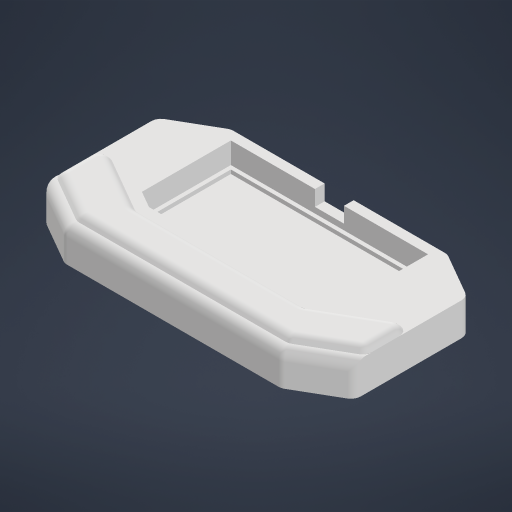
# Autodesk Inventor part: Joystick Bottom
Saved by Autodesk Inventor 2023.4 (Build 274418000, 418)
## iProperties
Created: 2024-04-17
Part Number: Joystick Bottom
Material: Generic
Document SubType Name: Modeling
Designer: xSibe
Density: 1 g/cm^3
Appearance: Default
Author: xSibe
Autodesk Inventor part; units mm, degrees
ref_plane "YZ Plane" through (0, 0, 0) normal (1, 0, 0) x (0, 1, 0)
ref_plane "XZ Plane" through (0, 0, 0) normal (0, 1, 0) x (-1, 0, 0)
ref_plane "XY Plane" through (0, 0, 0) normal (0, 0, 1) x (1, 0, 0)
sketch "Sketch1" plane through (0, 0, 0) normal (0, 1, 0) x (-1, 0, 0)
  line L0 (25.5, 11.5) -> (-25.5, 11.5)
  line L1 (-25.5, 11.5) -> (-25.5, -11.5)
  line L2 (-25.5, -11.5) -> (25.5, -11.5)
  line L3 (25.5, -11.5) -> (25.5, 11.5)
  line L4 (25.5, 11.5) -> (-25.5, -11.5) construction
  line L5 (-25.5, 11.5) -> (25.5, -11.5) construction
  line L6 (24.5, -10.5) -> (-24.5, -10.5)
  line L7 (-24.5, -10.5) -> (-24.5, 10.5)
  line L8 (-24.5, 10.5) -> (24.5, 10.5)
  line L9 (24.5, 10.5) -> (24.5, -10.5)
  line L10 (28, -14) -> (-28, -14)
  line L11 (-28, -14) -> (-28, 14)
  line L12 (-28, 14) -> (28, 14)
  line L13 (28, 14) -> (28, -14)
  line L14 (28, -14) -> (15.875644, -7)
  line L15 (15.875644, -7) -> (15.875644, 7)
  line L16 (15.875644, 7) -> (28, 14)
  line L17 (28, 14) -> (40.124356, 7)
  line L18 (40.124356, 7) -> (40.124356, -7)
  line L19 (40.124356, -7) -> (28, -14)
  line L20 (-28, -14) -> (-40.124356, -7)
  line L21 (-40.124356, -7) -> (-40.124356, 7)
  line L22 (-40.124356, 7) -> (-28, 14)
  line L23 (-28, 14) -> (-15.875644, 7)
  line L24 (-15.875644, 7) -> (-15.875644, -7)
  line L25 (-15.875644, -7) -> (-28, -14)
  line L26 (40.124356, 7) -> (40.124356, 22)
  line L27 (-28, 29) -> (28, 29)
  line L28 (-40.124356, 22) -> (-28, 29)
  line L29 (-40.124356, 22) -> (-40.124356, 7)
  line L30 (40.124356, 22) -> (28, 29)
  line L31 (28, 14) -> (28, 29)
  line L32 (-28, 14) -> (-28, 29)
  line L33 (-21.169873, 14) -> (21.169873, 14)
  line L34 (-25.5, 11.5) -> (-21.169873, 14)
  line L35 (25.5, 11.5) -> (21.169873, 14)
  point P0 (0, 0)
  point P1 (28, 0)
  point P2 (-28, 0)
  dimension "d0" = 51
  dimension "d1" = 23
  dimension "d2" = 1
  dimension "d3" = 2.5
  dimension "d13" = 15
  dimension "d20" = 15
  dimension "d21" = 90
  dimension "d22" = 60
  dimension "d23" = 150
  dimension "d24" = 150
  constraints: 72 end point, 7 parallel, 4 midpoint, 3 perpendicular, 3 vertical, 2 horizontal, 1 coincident, 1 collinear, 32 other
  measures "d0" distance of L2.end L1.end
  measures "d1" distance of L1.end L0.end
  measures "d2" distance between parallel lines of L2 L6
  measures "d3" distance between parallel lines of L2 L10
  measures "d13" distance of L17.end L26.end
  measures "d20" distance of L28.start L21.end
  measures "d21" angle of L31 L27
  measures "d22" angle of L28 L32
  measures "d23" angle of L33 L35
  measures "d24" angle of L34 L33
extrude "Extrusion1" add sketch "Sketch1" along normal blind 3
extrude "Extrusion2" cut sketch "Sketch1" against normal blind 1 from surface at 3 contours L16 L15 L14 L6 L25 L24 L23 L8 | L8 L9 L6 L14 L15 L16 | L23 L24 L25 L6 L7 L8
extrude "Extrusion3" add sketch "Sketch1" along normal blind 5.5 from surface at 3 contours L35 L16 L13 L14 L2 L3 | L35 L12 L16 | L14 L10 L25 L2 | L17 L18 L19 L13 | L31 L30 L26 L17 | L12 L32 L27 L31 | L1 L2 L25 L11 L23 L34 | L23 L12 L34 | L11 L20 L21 L22 | L22 L29 L28 L32
sketch "Sketch2" plane through (-28, 8.5, 14) normal (0, 1, 0) x (1, 0, 0)
  line L0 (2.5, 25.5) -> (2.5, 2.5)
  line L1 (53.5, 25.5) -> (2.5, 25.5)
  line L2 (53.5, 2.5) -> (53.5, 25.5)
  line L3 (0, 28) -> (56, 28)
  line L4 (53.5, 25.5) -> (53.5, 28)
  line L5 (2.5, 25.5) -> (2.5, 28)
  line L6 (2.5, 26.75) -> (53.5, 26.75)
  line L7 (24.25, 25.5) -> (31.75, 25.5)
  line L8 (31.75, 25.5) -> (31.75, 28)
  line L9 (31.75, 28) -> (24.25, 28)
  line L10 (24.25, 28) -> (24.25, 25.5)
  line L11 (24.25, 25.5) -> (31.75, 28) construction
  line L12 (31.75, 25.5) -> (24.25, 28) construction
  line L13 (68.124356, 21) -> (68.124356, -8)
  line L14 (56, 28) -> (68.124356, 21)
  line L15 (-12.124356, 21) -> (0, 28)
  line L16 (-12.124356, -8) -> (-12.124356, 21)
  line L17 (0, -15) -> (-12.124356, -8)
  line L18 (56, -15) -> (0, -15)
  line L19 (68.124356, -8) -> (56, -15)
  line L20 (6.830127, 0) -> (49.169873, 0)
  line L21 (2.5, 2.5) -> (6.830127, 0)
  line L22 (49.169873, 0) -> (53.5, 2.5)
  line L23 (53.5, 2.5) -> (2.5, 2.5)
  point P0 (28, 14)
  point P1 (28, 26.75)
  dimension "d10" = 7.5
  constraints: 20 end point, 5 midpoint, 3 perpendicular, 3 point on line, 2 horizontal, 2 parallel
  measures "d10" distance of L9.end L8.end
extrude "Extrusion4" cut sketch "Sketch2" against normal blind 4 contours L10 L6 L8 L1 | L10 L3 L8 L6
fillet "Fillet1" radius 2.5 11 edges at (-34.0622, 8.5, 25.5) (0, 8.5, 29) (34.0622, 8.5, 25.5) (40.1244, 4.25, 22) (28, 4.25, 29) (-28, 4.25, 29) (-40.1244, 4.25, 22) (-40.1244, 4.25, -7) (-28, 4.25, -14) (40.1244, 4.25, -7) (28, 4.25, -14)
extrude "Extrusion5" add sketch "Sketch2" along normal blind 3 from surface at -5.5 contours L23 L22 L20 L21
chamfer "Chamfer1" distance 1.675 angle 45 1 edges at (0, 6, 11.5)
sketch "Sketch3" plane through (-21.169873, 8.5, 14) normal (0, 1, 0) x (1, 0, 0)
  arc A0 (-1.25, -2.165064) -> (0, -2.5) centre (0, 0) ccw
  line L0 (0, -2.5) -> (42.339746, -2.5)
  arc A1 (42.339746, -2.5) -> (43.589746, -2.165064) centre (42.339746, 0) ccw
  line L1 (43.589746, -2.165064) -> (60.044229, 7.334936)
  arc A2 (60.044229, 7.334936) -> (61.294229, 9.5) centre (58.794229, 9.5) ccw
  line L2 (61.294229, 9.5) -> (61.294229, 19.556624)
  arc A3 (61.294229, 19.556624) -> (60.044229, 21.721688) centre (58.794229, 19.556624) ccw
  line L3 (60.044229, 21.721688) -> (49.75, 27.665064)
  arc A4 (49.75, 27.665064) -> (48.5, 28) centre (48.5, 25.5) ccw
  line L4 (48.5, 28) -> (-6.160254, 28)
  arc A5 (-6.160254, 28) -> (-7.410254, 27.665064) centre (-6.160254, 25.5) ccw
  line L5 (-7.410254, 27.665064) -> (-17.704483, 21.721688)
  arc A6 (-17.704483, 21.721688) -> (-18.954483, 19.556624) centre (-16.454483, 19.556624) ccw
  line L6 (-18.954483, 19.556624) -> (-18.954483, 9.5)
  arc A7 (-18.954483, 9.5) -> (-17.704483, 7.334936) centre (-16.454483, 9.5) ccw
  line L7 (-17.704483, 7.334936) -> (-1.25, -2.165064)
  line L8 (0.169873, 23.5) -> (42.169873, 23.5)
  arc A8 (44.669873, 21) -> (42.169873, 23.5) centre (42.169873, 21) ccw
  line L9 (44.669873, 21) -> (44.669873, 5.098076)
  arc A9 (43.419873, 2.933013) -> (44.669873, 5.098076) centre (42.169873, 5.098076) ccw
  line L10 (43.419873, 2.933013) -> (42.383975, 2.334936)
  arc A10 (41.133975, 2) -> (42.383975, 2.334936) centre (41.133975, 4.5) ccw
  line L11 (41.133975, 2) -> (28.044873, 2)
  arc A11 (-0.044229, 2.334936) -> (1.205771, 2) centre (1.205771, 4.5) ccw
  line L12 (-0.044229, 2.334936) -> (-1.080127, 2.933013)
  arc A12 (-2.330127, 5.098076) -> (-1.080127, 2.933013) centre (0.169873, 5.098076) ccw
  line L13 (-2.330127, 5.098076) -> (-2.330127, 21)
  arc A13 (0.169873, 23.5) -> (-2.330127, 21) centre (0.169873, 21) ccw
  arc A14 (49.75, 27.665064) -> (48.5, 28) centre (48.5, 25.5) ccw
  line L14 (60.044229, 21.721688) -> (49.75, 27.665064)
  arc A15 (61.294229, 19.556624) -> (60.044229, 21.721688) centre (58.794229, 19.556624) ccw
  line L15 (61.294229, -6.556624) -> (61.294229, 19.556624)
  arc A16 (60.044229, -8.721688) -> (61.294229, -6.556624) centre (58.794229, -6.556624) ccw
  line L16 (49.75, -14.665064) -> (60.044229, -8.721688)
  arc A17 (48.5, -15) -> (49.75, -14.665064) centre (48.5, -12.5) ccw
  line L17 (-6.160254, -15) -> (48.5, -15)
  arc A18 (-7.410254, -14.665064) -> (-6.160254, -15) centre (-6.160254, -12.5) ccw
  line L18 (-17.704483, -8.721688) -> (-7.410254, -14.665064)
  arc A19 (-18.954483, -6.556624) -> (-17.704483, -8.721688) centre (-16.454483, -6.556624) ccw
  line L19 (-18.954483, 19.556624) -> (-18.954483, -6.556624)
  arc A20 (-17.704483, 21.721688) -> (-18.954483, 19.556624) centre (-16.454483, 19.556624) ccw
  line L20 (-7.410254, 27.665064) -> (-17.704483, 21.721688)
  arc A21 (-6.160254, 28) -> (-7.410254, 27.665064) centre (-6.160254, 25.5) ccw
  line L21 (48.5, 28) -> (-6.160254, 28)
  line L22 (42.339746, -2.75) -> (0, -2.75)
  arc A22 (-1.375, -2.38157) -> (0, -2.75) centre (0, 0) ccw
  line L23 (-1.375, -2.38157) -> (-17.829483, 7.11843)
  arc A23 (-19.204483, 9.5) -> (-17.829483, 7.11843) centre (-16.454483, 9.5) ccw
  line L24 (-19.204483, 9.5) -> (-19.204483, 19.556624)
  arc A24 (-17.829483, 21.938194) -> (-19.204483, 19.556624) centre (-16.454483, 19.556624) ccw
  line L25 (-17.829483, 21.938194) -> (-7.535254, 27.88157)
  arc A25 (-6.160254, 28.25) -> (-7.535254, 27.88157) centre (-6.160254, 25.5) ccw
  line L26 (-6.160254, 28.25) -> (48.5, 28.25)
  arc A26 (49.875, 27.88157) -> (48.5, 28.25) centre (48.5, 25.5) ccw
  line L27 (49.875, 27.88157) -> (60.169229, 21.938194)
  arc A27 (61.544229, 19.556624) -> (60.169229, 21.938194) centre (58.794229, 19.556624) ccw
  line L28 (61.544229, 19.556624) -> (61.544229, 9.5)
  arc A28 (60.169229, 7.11843) -> (61.544229, 9.5) centre (58.794229, 9.5) ccw
  line L29 (60.169229, 7.11843) -> (43.714746, -2.38157)
  arc A29 (42.339746, -2.75) -> (43.714746, -2.38157) centre (42.339746, 0) ccw
  arc A30 (49.75, 27.665064) -> (48.5, 28) centre (48.5, 25.5) ccw
  line L30 (24.919873, 28) -> (48.5, 28)
  line L31 (24.919873, 28) -> (24.919873, 25.5)
  line L32 (46.669873, 25.5) -> (24.919873, 25.5)
  line L33 (46.669873, 2.5) -> (46.669873, 25.5)
  line L34 (42.339746, 0) -> (46.669873, 2.5)
  line L35 (0, 0) -> (42.339746, 0)
  line L36 (-4.330127, 2.5) -> (0, 0)
  line L37 (-4.330127, 25.5) -> (-4.330127, 2.5)
  line L38 (17.419873, 25.5) -> (-4.330127, 25.5)
  line L39 (17.419873, 25.5) -> (17.419873, 28)
  line L40 (-6.160254, 28) -> (17.419873, 28)
  arc A31 (-6.160254, 28) -> (-7.410254, 27.665064) centre (-6.160254, 25.5) ccw
  line L41 (-17.704483, 21.721688) -> (-7.410254, 27.665064)
  arc A32 (-17.704483, 21.721688) -> (-18.954483, 19.556624) centre (-16.454483, 19.556624) ccw
  line L42 (-18.954483, -5.113249) -> (-18.954483, 19.556624)
  line L43 (-6.160254, -12.5) -> (-18.954483, -5.113249)
  line L44 (48.5, -12.5) -> (-6.160254, -12.5)
  line L45 (61.294229, -5.113249) -> (48.5, -12.5)
  line L46 (61.294229, 19.556624) -> (61.294229, -5.113249)
  arc A33 (61.294229, 19.556624) -> (60.044229, 21.721688) centre (58.794229, 19.556624) ccw
  line L47 (49.75, 27.665064) -> (60.044229, 21.721688)
  arc A34 (27.294873, 2.75) -> (28.044873, 2) centre (28.044873, 2.75) ccw
  line L48 (27.294873, 2.75) -> (27.294873, 9)
  arc A35 (27.294873, 9) -> (23.544873, 9) centre (25.419873, 9) ccw
  line L49 (23.544873, 9) -> (23.544873, 2.75)
  arc A36 (22.794873, 2) -> (23.544873, 2.75) centre (22.794873, 2.75) ccw
  line L50 (22.794873, 2) -> (22.044873, 2)
  arc A37 (21.294873, 2.75) -> (22.044873, 2) centre (22.044873, 2.75) ccw
  line L51 (21.294873, 2.75) -> (21.294873, 9)
  arc A38 (21.294873, 9) -> (17.544873, 9) centre (19.419873, 9) ccw
  line L52 (17.544873, 9) -> (17.544873, 2.75)
  arc A39 (16.794873, 2) -> (17.544873, 2.75) centre (16.794873, 2.75) ccw
  line L53 (16.794873, 2) -> (1.205771, 2)
  point P0 (21.169873, 14)
  point P1 (-18.954483, 8.354356)
  point P2 (61.294229, 8.354356)
  dimension "d31" = 0.25
  constraints: 16 end point, 16 point on circle, 8 centre point, 15 other
  measures "d31" distance between parallel lines of L0 L22
extrude "Extrusion6" add sketch "Sketch3" along normal blind 1.25 contours A23 L23 A22 L22 A29 L29 A28 L15 L45 L44 L43 L19
fillet "Fillet2" radius 2.5 6 edges at (-40.1244, 9.125, 5.6456) (40.1244, 9.125, 5.6456) (40.1244, 9.125, 19.1132) (27.3301, 9.125, 26.5) (-27.3301, 9.125, 26.5) (-40.1244, 9.125, 19.1132)
chamfer "Chamfer2" distance 1.25 angle 45 16 edges at (-29.4596, 9.75, 12.3893) (-38.8744, 9.75, 8.3971) (-40.1244, 9.75, 14.116) (-39.7894, 9.75, 18.9199) (-33.3923, 9.75, 23) (-27.3073, 9.75, 26.4148) (0, 9.75, 26.5) (27.3073, 9.75, 26.4148) (33.3923, 9.75, 23) (39.7894, 9.75, 18.9199) (40.1244, 9.75, 14.116) (38.8744, 9.75, 8.3971) (29.4596, 9.75, 12.3893) (21.8816, 9.75, 16.6563) (0, 9.75, 16.75) (-21.8816, 9.75, 16.6563)
fillet "Fillet3" radius 2.5 16 edges at (-26.9838, 9.75, 25.2075) (-32.7674, 9.75, 21.9176) (-38.707, 9.75, 18.2949) (-38.8745, 9.75, 14.116) (-38.2494, 9.75, 9.4796) (-30.0846, 9.75, 13.4718) (-22.2051, 9.75, 17.8636) (0, 9.75, 17.9999) (22.2051, 9.75, 17.8636) (30.0846, 9.75, 13.4718) (38.2494, 9.75, 9.4796) (38.8745, 9.75, 14.116) (38.707, 9.75, 18.2949) (32.7674, 9.75, 21.9176) (26.9838, 9.75, 25.2075) (0, 9.75, 25.2501)
sketch "Sketch4" plane through (0, 0, 0) normal (0, -1, 0) x (1, 0, 0)
  arc A0 (27.330127, -14) -> (28.580127, -13.665064) centre (27.330127, -11.5) ccw
  line L0 (38.874356, -7.721688) -> (28.580127, -13.665064)
  arc A1 (38.874356, -7.721688) -> (40.124356, -5.556624) centre (37.624356, -5.556624) ccw
  line L1 (40.124356, 20.556624) -> (40.124356, -5.556624)
  arc A2 (40.124356, 20.556624) -> (38.874356, 22.721688) centre (37.624356, 20.556624) ccw
  line L2 (28.580127, 28.665064) -> (38.874356, 22.721688)
  arc A3 (28.580127, 28.665064) -> (27.330127, 29) centre (27.330127, 26.5) ccw
  line L3 (-27.330127, 29) -> (27.330127, 29)
  arc A4 (-27.330127, 29) -> (-28.580127, 28.665064) centre (-27.330127, 26.5) ccw
  line L4 (-38.874356, 22.721688) -> (-28.580127, 28.665064)
  arc A5 (-38.874356, 22.721688) -> (-40.124356, 20.556624) centre (-37.624356, 20.556624) ccw
  line L5 (-40.124356, -5.556624) -> (-40.124356, 20.556624)
  arc A6 (-40.124356, -5.556624) -> (-38.874356, -7.721688) centre (-37.624356, -5.556624) ccw
  line L6 (-28.580127, -13.665064) -> (-38.874356, -7.721688)
  arc A7 (-28.580127, -13.665064) -> (-27.330127, -14) centre (-27.330127, -11.5) ccw
  line L7 (27.330127, -14) -> (-27.330127, -14)
  line L8 (24.9, 28.9) -> (-24.9, 28.9)
  line L9 (-24.9, 28.9) -> (-24.9, -20.9)
  line L10 (-24.9, -20.9) -> (24.9, -20.9)
  line L11 (24.9, -20.9) -> (24.9, 28.9)
  line L12 (24.9, 28.9) -> (-24.9, -20.9) construction
  line L13 (-24.9, 28.9) -> (24.9, -20.9) construction
  line L14 (17.05, 21.05) -> (-17.05, 21.05)
  line L15 (-17.05, 21.05) -> (-17.05, -13.05)
  line L16 (-17.05, -13.05) -> (17.05, -13.05)
  line L17 (17.05, -13.05) -> (17.05, 21.05)
  line L18 (24.9, -20.9) -> (21.9, -20.9)
  line L19 (21.9, -20.9) -> (21.9, -17.9)
  line L20 (21.9, -17.9) -> (24.9, -17.9)
  line L21 (24.9, -17.9) -> (24.9, -20.9)
  circle A8 centre (21.9, -17.9) radius 1.875
  circle A9 centre (21.9, -17.9) radius 2.10625
  circle A10 centre (21.9, -17.9) radius 2.78125
  line L22 (24.9, -20.9) -> (14.4, -20.9)
  line L23 (14.4, -20.9) -> (14.4, -10.4)
  line L24 (14.4, -10.4) -> (24.9, -10.4)
  line L25 (24.9, -10.4) -> (24.9, -20.9)
  line L26 (24.9, -10.4) -> (20.8, -10.4)
  circle A11 centre (20.8, -10.4) radius 2.0725
  circle A12 centre (14.4, -16.8) radius 2.0725
  line L27 (24.9, -20.9) -> (17.05, -20.9)
  line L28 (17.05, -20.9) -> (17.05, -18.55)
  line L29 (22.55, -13.05) -> (24.9, -13.05)
  line L30 (24.9, -13.05) -> (24.9, -20.9)
  line L31 (22.55, -13.05) -> (17.05, -18.55)
  circle A13 centre (21.9, 25.9) radius 2.78125
  circle A14 centre (21.9, 25.9) radius 2.10625
  circle A15 centre (21.9, 25.9) radius 1.875
  circle A16 centre (14.4, 24.8) radius 2.0725
  circle A17 centre (20.8, 18.4) radius 2.0725
  line L32 (17.05, 26.55) -> (22.55, 21.05)
  line L33 (24.9, 21.05) -> (22.55, 21.05)
  line L34 (17.05, 26.55) -> (17.05, 28.9)
  circle A18 centre (-21.9, 25.9) radius 2.78125
  circle A19 centre (-21.9, 25.9) radius 2.10625
  circle A20 centre (-21.9, 25.9) radius 1.875
  circle A21 centre (-20.8, 18.4) radius 2.0725
  circle A22 centre (-14.4, 24.8) radius 2.0725
  line L35 (-22.55, 21.05) -> (-17.05, 26.55)
  line L36 (-17.05, 28.9) -> (-17.05, 26.55)
  line L37 (-22.55, 21.05) -> (-24.9, 21.05)
  circle A23 centre (-21.9, -17.9) radius 2.78125
  circle A24 centre (-21.9, -17.9) radius 2.10625
  circle A25 centre (-21.9, -17.9) radius 1.875
  circle A26 centre (-14.4, -16.8) radius 2.0725
  circle A27 centre (-20.8, -10.4) radius 2.0725
  line L38 (-17.05, -18.55) -> (-22.55, -13.05)
  line L39 (-24.9, -13.05) -> (-22.55, -13.05)
  line L40 (-17.05, -18.55) -> (-17.05, -20.9)
  line L41 (17.05, -18.55) -> (-17.05, -18.55)
  line L42 (-22.55, -13.05) -> (-22.55, 21.05)
  line L43 (-17.05, 26.55) -> (17.05, 26.55)
  line L44 (22.55, 21.05) -> (22.55, -13.05)
  line L45 (0, 29) -> (0, 4)
  point P0 (-145.320015, 0.346167)
  point P1 (-153.170015, 8.196167)
  point P2 (-187.270015, 8.196167)
  point P3 (-195.120015, 0.346167)
  point P4 (-195.120015, -33.753833)
  point P5 (-187.270015, -41.603833)
  point P6 (-145.320015, -33.753833)
  point P7 (-153.170015, -41.603833)
  point P8 (-185.730311, -39.253833)
  point P9 (-155.820015, -41.603833)
  point P10 (-155.820015, -39.576333)
  point P11 (-156.930311, -39.253833)
  point P12 (-183.50972, -39.253833)
  point P13 (-192.770015, -32.214128)
  point P14 (-192.770015, -29.993537)
  point P15 (-192.770015, -3.414128)
  point P16 (-192.770015, -1.193537)
  point P17 (-185.730311, 5.846167)
  point P18 (-183.50972, 5.846167)
  point P19 (-156.930311, 5.846167)
  point P20 (-154.70972, 5.846167)
  point P21 (-147.670015, -32.214128)
  point P22 (-147.670015, -1.193537)
  point P23 (-147.670015, -3.414128)
  point P24 (-147.670015, -29.993537)
  point P25 (-154.70972, -39.253833)
  dimension "d41" = 49.8
  dimension "d42" = 49.8
  dimension "d43" = 7.85
  dimension "d44" = 3
  dimension "d45" = 3
  dimension "d46" = 3.75
  dimension "d47" = 4.2125
  dimension "d48" = 0.675
  dimension "d49" = 10.5
  dimension "d50" = 10.5
  dimension "d51" = 4.1
  dimension "d52" = 4.145
  dimension "d53" = 7.85
  dimension "d54" = 7.85
  dimension "d55" = 5.5
  dimension "d56" = 5.5
  dimension "d57" = 360
  dimension "d60" = 25
  constraints: 76 end point, 20 centre point, 10 parallel, 8 coincident, 7 perpendicular, 4 horizontal, 3 midpoint, 3 point on line, 1 symmetric about line, 1 vertical, 69 other
  measures "d41" distance of L10.end L9.end
  measures "d42" distance of L9.end L8.end
  measures "d43" distance between parallel lines of L11 L17
  measures "d44" distance of L19.end L20.end
  measures "d45" distance of L18.end L19.end
  measures "d46" diameter of A8
  measures "d47" diameter of A9
  measures "d48" radial gap between concentric circles of A9 A10
  measures "d49" distance of L23.end L24.end
  measures "d50" distance of L22.end L23.end
  measures "d51" distance of L24.end L26.end
  measures "d52" diameter of A11
  measures "d53" distance of point (17.05, -13.05) L29.end
  measures "d54" distance of L27.end point (17.05, -13.05)
  measures "d55" distance of L29.start point (17.05, -13.05)
  measures "d56" distance of L28.end point (17.05, -13.05)
  measures "d60" distance of L45.start L45.end
extrude "Extrusion7" cut sketch "Sketch4" against normal blind 2 contours L44 A17 | A17 L44 | L43 A16 | A16 L43 | L42 A21 | A21 L42 | L43 A22 | A22 L43
body "Solid1"
